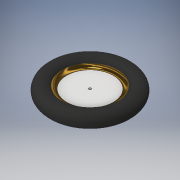
# Autodesk Inventor part: wheel
Saved by Autodesk Inventor 2019 (Build 230136000, 136)
## iProperties
Created: 2018-08-20
Part Number: wheel
Material: Generic
Document SubType Name: Modeling
Designer: Kitte_X
Density: 1 g/cm^3
Appearance: Default
Author: Kitte_X
Autodesk Inventor part; units mm, degrees
ref_plane "YZ Plane" through (0, 0, 0) normal (1, 0, 0) x (0, 1, 0)
ref_plane "XZ Plane" through (0, 0, 0) normal (0, 1, 0) x (-1, 0, 0)
ref_plane "XY Plane" through (0, 0, 0) normal (0, 0, 1) x (1, 0, 0)
sketch "Sketch1" plane through (0, 0, 0) normal (1, 0, 0) x (0, 1, 0)
  line L0 (0, 0) -> (0, 165.1) construction
  arc A0 (14.4, 108.7819) -> (-14.4, 108.7819) centre (0, 135.1) ccw
  line L1 (4, 91.2366) -> (4, 5)
  line L2 (-4, 5) -> (-4, 91.2366)
  arc A1 (14.4, 108.7819) -> (4, 91.2366) centre (24, 91.2366) ccw
  arc A2 (-4, 91.2366) -> (-14.4, 108.7819) centre (-24, 91.2366) ccw
  line L3 (4, 5) -> (-4, 5)
  line L4 (-42, 0) -> (42, 0) projected
  point P0 (4, 105.3679)
  point P1 (-4, 105.3679)
  dimension "d0" = 165.1
  dimension "d1" = 60
  dimension "d2" = 4
  dimension "d3" = 4
  dimension "d4" = 20
  dimension "d5" = 5
  constraints: 9 point on circle, 8 end point, 4 tangent, 3 centre point, 3 point on line, 3 vertical, 1 equal radius, 1 perpendicular
  measures "d0" distance of L0.start L0.end
  measures "d1" diameter of A0
  measures "d2" distance between parallel lines of L2 L0
  measures "d3" distance between parallel lines of L0 L1
  measures "d4" radius of A1
  measures "d5" distance from line of L0.start L3
revolve "Revolution1" add sketch "Sketch1" angle 360 about axis through (0, -10, 0) along (0, 1, 0)
body "Solid1"
